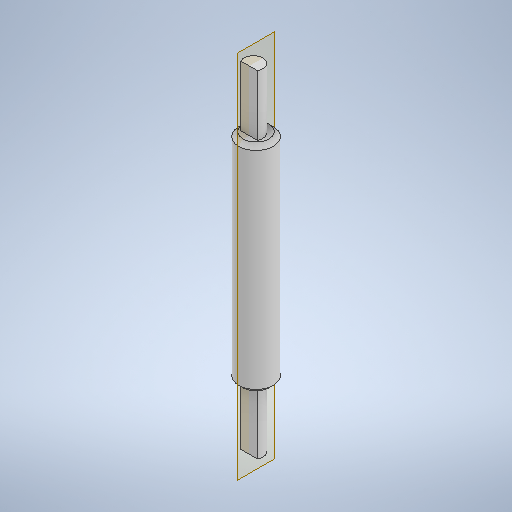
# Autodesk Inventor part: axle-skibidi
Saved by Autodesk Inventor 2025 (Build 290162010, 162A)
## iProperties
Created: 2024-08-26
Part Number: axle-skibidi
Material: Generic
Document SubType Name: Modeling
Designer: limfe
Density: 1 g/cm^3
Appearance: Default
Author: limfe
Autodesk Inventor part; units mm, degrees
ref_plane "XZ Plane" through (0, 0, 0) normal (0, 1, 0) x (-1, 0, 0)
ref_plane "XY Plane" through (0, 0, 0) normal (0, 0, 1) x (1, 0, 0)
sketch "Sketch1" plane through (0, 0, 0) normal (0, 1, 0) x (-1, 0, 0)
  circle A0 centre (0, 0) radius 2
  dimension "d0" = 4
  constraints: 2 coincident, 1 centre point
  measures "d0" diameter of A0
extrude "Extrusion1" add sketch "Sketch1" along normal blind 25
sketch "Sketch2" plane through (0, 25, 0) normal (0, 1, 0) x (1, 0, 0)
  line L0 (0, -2) -> (2.3553, -2)
  line L1 (-0.9798, -0.8) -> (0.9798, -0.8)
  arc A0 (0.9798, -0.8) -> (-0.9798, -0.8) centre (0, -0.3) ccw
  circle A1 centre (0, 0) radius 2 projected
  line L2 (3.2263, 0) -> (-2.8711, 0) projected
  dimension "d4" = 1.2
  dimension "d6" = 1.1
  dimension "d7" = 0.3
  constraints: 4 end point, 2 horizontal, 2 point on circle, 1 centre point, 1 tangent, 1 vertical alignment
  measures "d4" distance between parallel lines of L0 L1
  measures "d6" radius of A0
  measures "d7" distance from line of A0.centre L2
extrude "Extrusion2" add sketch "Sketch2" along normal blind 7 contours A0 L2 L1 | A0 L2
sketch "Sketch3" plane through (0, 0, 0) normal (0, -1, 0) x (1, 0, 0)
  line L0 (-0.9798, 0.8) -> (0.9798, 0.8)
  arc A0 (-0.9798, 0.8) -> (0.9798, 0.8) centre (0, 0.3) ccw
  point P0 (0, 0)
  point P1 (0, 0)
  point P2 (0, 0.8)
  dimension "d12" = 1.9596
  dimension "d16" = 1.1
  dimension "d17" = 0.3
  constraints: 2 coincident, 2 end point, 2 point on circle, 1 centre point, 1 horizontal, 1 midpoint, 1 vertical alignment
  measures "d12" distance of L0.start L0.end
  measures "d16" radius of A0
  measures "d17" distance of point (0, 0) A0.centre
extrude "Extrusion3" add sketch "Sketch3" along normal blind 7
chamfer "Chamfer1" distance 0.5 angle 45 1 edges at (2, 25, 0)
chamfer "Chamfer2" distance 0.5 angle 45 1 edges at (2, 0, 0)
equation "\"d4\" = d3"
equation "\"d3\" = 1.2"
body "Solid1"
